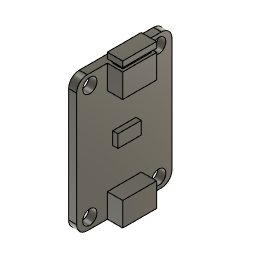
VL53L0X+ToF+Sensor (Autodesk Fusion 360 design; units mm, degrees)
Autodesk Fusion 360 part; units mm, degrees
sketch "Sketch1" plane through (0, 0, 0) normal (1, 0, 0) x (0, 1, 0)
  line L0 (0, 0) -> (18, 0)
  line L1 (18, 0) -> (18, 25.5)
  line L2 (18, 25.5) -> (0, 25.5)
  line L3 (0, 25.5) -> (0, 0)
  line L4 (5.8, 25.5) -> (12.2, 25.5)
  line L5 (12.2, 25.5) -> (12.2, 21)
  line L6 (12.2, 21) -> (5.8, 21)
  line L7 (5.8, 21) -> (5.8, 25.5)
  line L8 (9, 0) -> (9, 25.5)
  line L9 (12.2, 23.25) -> (9, 23.25)
  line L10 (5.8, 23.25) -> (9, 23.25)
  line L11 (0, 12.75) -> (18, 12.75)
  line L12 (5.8, 4.5) -> (5.8, 0)
  line L13 (5.8, 0) -> (12.2, 0)
  line L14 (12.2, 0) -> (12.2, 4.5)
  line L15 (12.2, 4.5) -> (5.8, 4.5)
  line L16 (6.8, 13.95) -> (11.2, 13.95)
  line L17 (11.2, 13.95) -> (11.2, 11.55)
  line L18 (11.2, 11.55) -> (6.8, 11.55)
  line L19 (6.8, 11.55) -> (6.8, 13.95)
  line L20 (8, 13.95) -> (8, 12.75)
  line L21 (8, 11.55) -> (8, 12.75)
  line L22 (11.2, 13.3189) -> (9, 13.3189)
  line L23 (6.8, 13.3189) -> (9, 13.3189)
  dimension "d1" = 25.5
  dimension "d2" = 18
  dimension "d3" = 6.4
  dimension "d4" = 4.5
  dimension "d5" = 4.4
  dimension "d6" = 2.4
  constraint horizontal L0
  constraint vertical L1
  constraint horizontal L2
  constraint vertical L3
  constraint coincident L0.start L3.end
  constraint horizontal L4
  constraint vertical L5
  constraint horizontal L6
  constraint vertical L7
  constraint coincident L2 L4.start
  constraint midpoint L0 L8.start
  constraint midpoint L2 L8.end
  constraint midpoint L5 L9.start
  constraint coincident L8 L9.end
  constraint perpendicular L8 L9
  constraint midpoint L7 L10.start
  constraint equal L9 L10
  constraint midpoint L3 L11.start
  constraint midpoint L1 L11.end
  constraint symmetric L4.start L11 L12.end
  constraint symmetric L4.end L11 L13.end
  constraint symmetric L5.end L11 L14.end
  constraint symmetric L6.end L11 L12.start
  constraint horizontal L16
  constraint vertical L17
  constraint horizontal L18
  constraint vertical L19
  constraint coincident L16 L20.start
  constraint coincident L11 L20.end
  constraint perpendicular L11 L20
  constraint coincident L18 L21.start
  constraint perpendicular L11 L21
  constraint equal L20 L21
  constraint coincident L17 L22.start
  constraint coincident L8 L22.end
  constraint perpendicular L8 L22
  constraint coincident L19 L23.start
  constraint perpendicular L8 L23
  constraint equal L22 L23
  measures "d1" distance of L0.start L2.end
  measures "d2" distance of L0.start L0.end
  measures "d3" distance of L5 L7
  measures "d4" distance of L4.end L5.end
  measures "d5" distance of L16.start L16.end
  measures "d6" distance of L16.start L18.end
extrude "Extrude1" add sketch "Sketch1" against normal blind 1.5
extrude "Extrude2" add sketch "Sketch1" along normal blind 2.9 contours L0 L8 L12 L13 L15 | L0 L8 L13 L14 L15 | L2 L4 L7 L8 L10 | L2 L4 L5 L8 L9 | L6 L7 L8 L10 | L5 L6 L8 L9
extrude "Extrude3" add sketch "Sketch1" along normal blind 1 contours L11 L19 L20 L23 | L11 L18 L19 L21 | L8 L11 L20 L23 | L8 L11 L18 L21 | L16 L19 L20 L23 | L8 L11 L17 L18 | L8 L11 L17 L22 | L8 L16 L20 L23 | L8 L16 L17 L22
sketch "Sketch2" plane through (0, 0, 25.5) normal (0, 0, 1) x (-1, 0, 0)
  line L0 (0, -12.2) -> (0, -18)
  line L1 (0, -18) -> (1.5, -18)
  line L2 (1.5, -18) -> (1.5, 0)
  line L3 (1.5, 0) -> (0, 0)
  line L4 (0, 0) -> (0, -5.8)
  line L5 (0, -5.8) -> (-2.9, -5.8)
  line L6 (-2.9, -5.8) -> (-2.9, -12.2)
  line L7 (-2.9, -12.2) -> (0, -12.2)
  line L8 (-2.4, -6.3) -> (-0.5, -6.3)
  line L9 (-0.5, -6.3) -> (-0.5, -11.7)
  line L10 (-0.5, -11.7) -> (-2.4, -11.7)
  line L11 (-2.4, -11.7) -> (-2.4, -6.3)
  line L12 (0, -5.8) -> (0, -12.2)
  dimension "d13" = 0.5
  dimension "d14" = 0.5
  dimension "d15" = 0.5
  dimension "d16" = 0.5
  constraint horizontal L8
  constraint vertical L9
  constraint horizontal L10
  constraint vertical L11
  measures "d13" distance of L5 L8
  measures "d14" distance of L6 L11
  measures "d15" distance of L9 L12
  measures "d16" distance of L7 L10
extrude "Extrude4" add sketch "Sketch2" along normal blind 0.7 contours L8 L9 L10 L11
sketch "Sketch3" plane through (0, 0, 26.2) normal (0, 0, 1) x (-1, 0, 0)
  line L0 (-2.4, -11.7) -> (-0.5, -11.7)
  line L1 (-0.5, -11.7) -> (-0.5, -6.3)
  line L2 (-0.5, -6.3) -> (-2.4, -6.3)
  line L3 (-2.4, -6.3) -> (-2.4, -11.7)
  line L4 (-2.4, -11.7) -> (-2.4, -6.3)
  line L5 (-2.4, -6.3) -> (-0.5, -6.3)
  line L6 (-0.5, -6.3) -> (-0.5, -11.7)
  line L7 (-0.5, -11.7) -> (-2.4, -11.7)
  line L8 (0, -12.2) -> (0, -18)
  line L9 (0, -18) -> (1.5, -18)
  line L10 (1.5, -18) -> (1.5, 0)
  line L11 (1.5, 0) -> (0, 0)
  line L12 (0, 0) -> (0, -5.8)
  line L13 (0, -5.8) -> (-2.9, -5.8)
  line L14 (-2.9, -5.8) -> (-2.9, -12.2)
  line L15 (-2.9, -12.2) -> (0, -12.2)
  line L16 (-2.9, -5.8) -> (0, -5.8)
  line L17 (0, -5.8) -> (0, -12.2)
  line L18 (0, -12.2) -> (-2.9, -12.2)
  line L19 (-2.9, -12.2) -> (-2.9, -5.8)
  constraint horizontal L16
  constraint vertical L17
  constraint horizontal L18
  constraint vertical L19
  constraint coincident L8.start L15.end
  constraint coincident L13.end L14.start
extrude "Extrude5" add sketch "Sketch3" along normal blind 1.1 contours L0 L1 L2 L3 L4 L5 L6 L7 | L13 L14 L15 L16 L17 L18 L19
sketch "Sketch4" plane through (0, 0, 0) normal (1, 0, 0) x (0, 1, 0)
  line L0 (6.8, 11.55) -> (6.8, 13.95)
  line L1 (6.8, 13.95) -> (11.2, 13.95)
  line L2 (11.2, 13.95) -> (11.2, 11.55)
  line L3 (11.2, 11.55) -> (6.8, 11.55)
  line L4 (12.2, 25.5) -> (12.2, 21)
  line L5 (12.2, 21) -> (5.8, 21)
  line L6 (5.8, 21) -> (5.8, 25.5)
  line L7 (5.8, 25.5) -> (0, 25.5)
  line L8 (0, 25.5) -> (0, 0)
  line L9 (0, 0) -> (5.8, 0)
  line L10 (5.8, 0) -> (5.8, 4.5)
  line L11 (5.8, 4.5) -> (12.2, 4.5)
  line L12 (12.2, 4.5) -> (12.2, 0)
  line L13 (12.2, 0) -> (18, 0)
  line L14 (18, 0) -> (18, 25.5)
  line L15 (18, 25.5) -> (12.2, 25.5)
  circle A0 centre (2.5, 23.5) radius 1.35
  line L16 (9, 13.95) -> (9, 20)
  line L17 (6.8, 12.75) -> (1, 12.75)
  circle A1 centre (15.5, 23.5) radius 1.35
  circle A2 centre (2.5, 2) radius 1.35
  circle A3 centre (15.5, 2) radius 1.35
  dimension "d22" = 2.7
  dimension "d23" = 2
  dimension "d24" = 2.5
  constraint midpoint L1 L16.start
  constraint perpendicular L5 L16
  constraint midpoint L0 L17.start
  constraint perpendicular L0 L17
  constraint symmetric A0 L16 A1
  constraint symmetric A0 L17 A2
  constraint symmetric L17 A1 A3
  measures "d22" diameter of A0
  measures "d23" distance of L7 A0.centre
  measures "d24" distance of L8 A0.centre
extrude "Extrude6" cut sketch "Sketch4" against normal blind 4 contours A0 | A1 | A2 | A3
fillet "Fillet1" radius 2 4 edges at (-0.75, 0, 25.5) (-0.75, 18, 25.5) (-0.75, 18, 0) (-0.75, 0, 0)
